holderright (Autodesk Fusion 360 design; units mm, degrees)
Autodesk Fusion 360 part; units mm, degrees
sketch "Sketch1" plane through (0, 0, 0) normal (0, 1, 0) x (1, 0, 0)
  line L0 (0, 0) -> (35, -80)
  line L1 (35, -80) -> (65, -80)
  line L2 (65, -80) -> (100, 0)
  line L3 (100, 0) -> (0, 0)
  circle A0 centre (50, -50) radius 7.5
  circle A1 centre (50, -50) radius 3
  dimension "d1" = 100
  dimension "d2" = 30
  dimension "d4" = 80
  dimension "d5" = 35
  dimension "d6" = 50
  dimension "d7" = 15
  dimension "d8" = 15
  dimension "d13" = 6
  constraint horizontal L1
  constraint parallel L1 L3
  constraint coincident L0.start L3.end
  constraint concentric A0 A1
  measures "d1" distance of L0.start L2.end
  measures "d2" distance of L0.end L1.end
  measures "d4" distance of L1 L3
  measures "d5" horizontal distance of L0.start L0.end
  measures "d6" vertical distance of L0.start A0.centre
  measures "d7" diameter of A0
  measures "d8" horizontal distance of L1.end A0.centre
  measures "d13" diameter of A1
extrude "Extrude1" add sketch "Sketch1" against normal blind 5 contours L0 L1 L2 L3 | A0 | A1
extrude "Extrude2" add sketch "Sketch1" along normal blind 34 contours A1
fillet "Fillet1" radius 9 2 edges at (65, -2.5, 80) (35, -2.5, 80)
